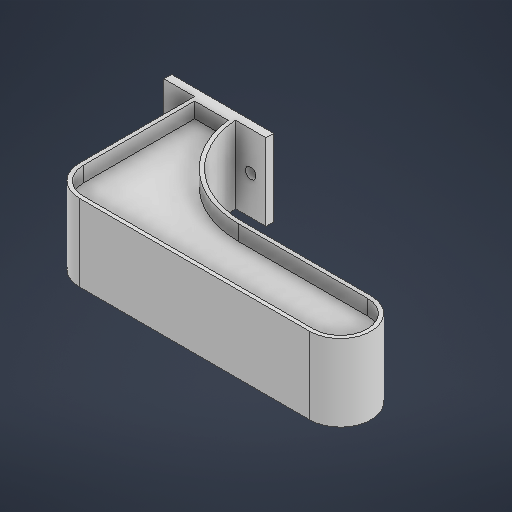
# Autodesk Inventor part: Pylon
Saved by Autodesk Inventor 2026.1 (Build 301233000, 233)
## iProperties
Created: 2025-09-15
Part Number: Pylon
Material: Generic
Document SubType Name: Modeling
Designer: mateo
Density: 1 g/cm^3
Appearance: Default
Author: mateo
Autodesk Inventor part; units mm, degrees
ref_plane "YZ Plane" through (0, 0, 0) normal (1, 0, 0) x (0, 1, 0)
ref_plane "XZ Plane" through (0, 0, 0) normal (0, 1, 0) x (-1, 0, 0)
ref_plane "XY Plane" through (0, 0, 0) normal (0, 0, 1) x (1, 0, 0)
sketch "Sketch1" plane through (0, 0, 0) normal (0, 1, 0) x (-1, 0, 0)
  line L0 (0, 0) -> (80, 0)
  line L1 (20, 5) -> (0, 5)
  line L2 (0, 5) -> (0, 0)
  line L3 (46.5184, 5) -> (46.5184, 80)
  circle A0 centre (26.5184, 80) radius 20
  line L4 (26.5184, 100) -> (-123.4816, 100)
  circle A1 centre (-123.4816, 80) radius 20
  line L5 (-123.4816, 60) -> (-39.7913, 60)
  arc A2 (20, 5) -> (-39.7913, 60) centre (-39.7913, 0) ccw
  line L6 (46.5184, 5) -> (66.5184, 5)
  line L7 (66.5184, 5) -> (66.5184, 0)
  line L8 (66.5184, 0) -> (46.5184, 0)
  point P0 (16.5184, 60)
  dimension "d1" = 75
  dimension "d2" = 40
  dimension "d3" = 150
  dimension "d4" = 140
  dimension "d7" = 40
  dimension "d10" = 5
  dimension "d11" = 5
  constraints: 18 end point, 6 point on circle, 4 horizontal, 3 centre point, 3 tangent, 2 parallel, 1 perpendicular, 1 point on line, 1 vertical
  measures "d1" distance of L3.start L3.end
  measures "d2" diameter of A0
  measures "d3" distance of L4.start L4.end
  measures "d4" distance of L5.start point (16.518, 60)
  measures "d7" diameter of A1
  measures "d10" distance of L6.end L7.end
  measures "d11" distance of L1.end L0.start
extrude "Extrusion1" add sketch "Sketch1" along normal blind 50
sketch "Sketch2" plane through (-20, 0, 5) normal (0, 0, 1) x (1, 0, 0)
  circle A0 centre (10, 25) radius 3.5
  line L0 (20, 0) -> (20, 50) projected
  line L1 (0, 50) -> (20, 50) projected
  circle A1 centre (-36.5184, 25) radius 3.5
  line L2 (-46.5184, 0) -> (-46.5184, 50) projected
  line L3 (-46.5184, 50) -> (-26.5184, 50) projected
  dimension "d14" = 7
  dimension "d15" = 10
  dimension "d16" = 25
  dimension "d17" = 7
  dimension "d18" = 10
  dimension "d22" = 25
  constraints: 2 centre point
  measures "d14" diameter of A0
  measures "d15" distance from line of L0 A0.centre
  measures "d16" distance from line of L1 A0.centre
  measures "d17" diameter of A1
  measures "d18" distance from line of A1.centre L2
  measures "d22" distance from line of A1.centre L3
extrude "Extrusion2" cut sketch "Sketch2" against normal blind 20
sketch "Sketch3" plane through (0, 50, 0) normal (0, 1, 0) x (1, 0, 0)
  line L0 (-46.5184, -5) -> (-46.5184, -80) projected
  arc A0 (-20, -5) -> (39.7913, -60) centre (39.7913, 0) ccw projected
  line L1 (-26.5184, -100) -> (123.4816, -100) projected
  arc A1 (123.4816, -100) -> (123.4816, -60) centre (123.4816, -80) ccw projected
  line L2 (123.4816, -60) -> (39.7913, -60) projected
  arc A2 (-20, -5) -> (39.7913, -60) centre (39.7913, 0) ccw projected
  line L3 (-46.5184, -5) -> (-46.5184, -80) projected
  arc A3 (-46.5184, -80) -> (-26.5184, -100) centre (-26.5184, -80) ccw projected
  arc A4 (-46.5184, -80) -> (-26.5184, -100) centre (-26.5184, -80) ccw projected
  line L4 (-46.5184, -5) -> (-20, -5)
  line L5 (-26.5184, -97.5) -> (123.4816, -97.5)
  arc A5 (123.4816, -97.5) -> (123.4816, -62.5) centre (123.4816, -80) ccw
  line L6 (123.4816, -62.5) -> (39.7913, -62.5)
  arc A6 (-22.2571, -7.5) -> (39.7913, -62.5) centre (39.7913, 0) ccw
  line L7 (-22.2571, -7.5) -> (-44.0184, -7.5)
  line L8 (-44.0184, -7.5) -> (-44.0184, -80)
  line L9 (-26.5184, -97.5) -> (123.4816, -97.5)
  arc A7 (123.4816, -97.5) -> (123.4816, -62.5) centre (123.4816, -80) ccw
  line L10 (123.4816, -62.5) -> (39.7913, -62.5)
  arc A8 (-22.2571, -7.5) -> (39.7913, -62.5) centre (39.7913, 0) ccw
  line L11 (-22.2571, -7.5) -> (-44.0184, -7.5)
  line L12 (-44.0184, -7.5) -> (-44.0184, -80)
  arc A9 (-44.0184, -80) -> (-26.5184, -97.5) centre (-26.5184, -80) ccw
  point P0 (0, 0)
  point P1 (39.7913, -60)
  dimension "d24" = 2.5
  dimension "d25" = 2.5
  constraints: 18 end point, 10 point on circle, 8 centre point, 11 other
  measures "d24" distance between parallel lines of L4 L7
  measures "d25" radial gap between concentric circles of A3 A9
extrude "Extrusion3" cut sketch "Sketch3" against normal blind 10 contours A9 L8 L7 A6 L6 A5 L5
sketch "Sketch4" plane through (0, 0, 0) normal (0, -1, 0) x (1, 0, 0)
  arc A0 (39.7913, 60) -> (-20, 5) centre (39.7913, 0) ccw projected
  line L0 (-20, 5) -> (-46.5184, 5)
  line L1 (-46.5184, 5) -> (-46.5184, 80) projected
  arc A1 (-26.5184, 100) -> (-46.5184, 80) centre (-26.5184, 80) ccw projected
  line L2 (123.4816, 60) -> (39.7913, 60) projected
  arc A2 (123.4816, 60) -> (123.4816, 100) centre (123.4816, 80) ccw projected
  line L3 (-26.5184, 100) -> (123.4816, 100) projected
  arc A3 (123.4816, 62.5) -> (123.4816, 97.5) centre (123.4816, 80) ccw
  line L4 (123.4816, 62.5) -> (39.7913, 62.5)
  arc A4 (39.7913, 62.5) -> (-22.2571, 7.5) centre (39.7913, 0) ccw
  line L5 (-22.2571, 7.5) -> (-44.0184, 7.5)
  line L6 (-44.0184, 7.5) -> (-44.0184, 80)
  arc A5 (-26.5184, 97.5) -> (-44.0184, 80) centre (-26.5184, 80) ccw
  line L7 (-26.5184, 97.5) -> (123.4816, 97.5)
  point P0 (0, 0)
  dimension "d28" = 2.5
  constraints: 10 end point, 6 point on circle, 3 centre point, 6 other
  measures "d28" distance between parallel lines of L3 L7
extrude "Extrusion4" cut sketch "Sketch4" against normal blind 10 contours L4 A4 L5 L6 A5 L7 A3
body "Solid1"
